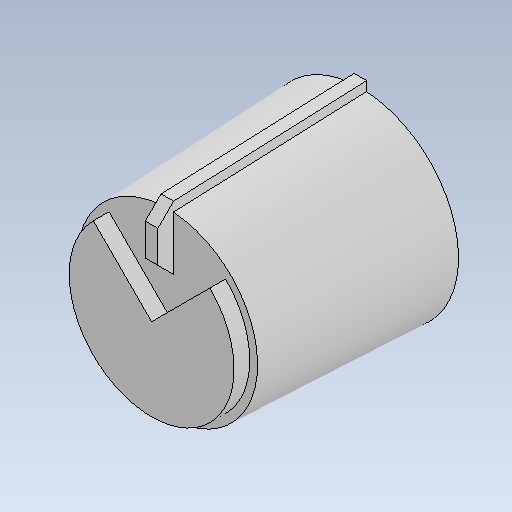
# Autodesk Inventor part: knob
Saved by Autodesk Inventor 2026.1 (Build 301233020, 233B)
## iProperties
Created: 2026-08-15
Part Number: knob
Material: 一般
Document SubType Name: Modeling
Designer: ug_nd
Density: 1 g/cm^3
Appearance: 既定
Author: ug_nd
Autodesk Inventor part; units mm, degrees
ref_plane "YZ Plane" through (0, 0, 0) normal (1, 0, 0) x (0, 1, 0)
ref_plane "XZ Plane" through (0, 0, 0) normal (0, 1, 0) x (-1, 0, 0)
ref_plane "XY Plane" through (0, 0, 0) normal (0, 0, 1) x (1, 0, 0)
sketch "スケッチ1" plane through (0, 0, 0) normal (1, 0, 0) x (0, 1, 0)
  line L0 (0, 0) -> (6.25, 0)
  line L1 (6.25, 0) -> (5.75, 12.3)
  line L2 (5.75, 12.3) -> (5.25, 12.3)
  line L3 (0, 13.3) -> (0, 0)
  line L4 (0, -2.66) -> (0, 15.96) construction
  line L5 (5.25, 12.3) -> (5.25, 13.3)
  line L6 (5.25, 13.3) -> (0, 13.3)
  dimension "d0" = 12.5
  dimension "d1" = 10.5
  dimension "d2" = 1
  dimension "d3" = 13.3
  dimension "d4" = 11.5
  constraints: 12 end point, 3 horizontal, 2 vertical, 2 other
  measures "d2" distance between parallel lines of L2 L6
  measures "d3" distance between parallel lines of L6 L0
revolve "回転1" add sketch "スケッチ1" angle 360 about axis through (0, 0, -10) along (0, 0, 1)
sketch "スケッチ2" plane through (0, 0, 13.3) normal (0, 0, 1) x (1, 0, 0)
  line L0 (0, -8.75) -> (0, 8.75) construction
  line L1 (0, 0) -> (3.7123, 3.7123)
  circle A0 centre (0, 0) radius 5.25 construction
  line L2 (0, 0) -> (-3.7123, 3.7123)
  arc A1 (3.7123, 3.7123) -> (-3.7123, 3.7123) centre (0, 0) ccw
  constraints: 4 end point, 2 point on circle, 1 centre point, 1 perpendicular, 1 symmetric about line, 3 other
extrude "押し出し1" cut sketch "スケッチ2" against normal up to surface (1 mm away)
sketch "スケッチ3" plane through (0, 0, 0) normal (1, 0, 0) x (0, 1, 0)
  line L0 (6.85, 0) -> (6.3093, 13.3)
  line L1 (6.3093, 13.3) -> (2.3093, 13.3)
  line L2 (6.25, 0) -> (-6.25, 0) construction
  line L3 (-6.25, 0) -> (-5.75, 12.3) construction
  line L4 (-5.75, 12.3) -> (-5.25, 12.3) construction
  line L5 (-5.25, 12.3) -> (-5.25, 13.3) construction
  line L6 (-5.25, 13.3) -> (0, 13.3) construction
  line L7 (0, 13.3) -> (0, 12.3) construction
  line L8 (0, 12.3) -> (5.75, 12.3) construction
  line L9 (5.75, 12.3) -> (6.25, 0) projected
  line L10 (6.85, 0) -> (6.25, 0)
  line L11 (2.3093, 13.3) -> (2.3093, 12.3)
  line L12 (5.75, 12.3) -> (2.3093, 12.3)
  line L13 (6.35, 12.3) -> (5.35, 13.3)
  line L14 (2.3093, 12.3) -> (3.3093, 13.3)
  point P0 (0, 0)
  dimension "d8" = 1
  dimension "d9" = 13.1
  dimension "d10" = 0.6
  dimension "d11" = 4
  dimension "d14" = 45
  constraints: 14 end point, 4 point on line, 2 horizontal, 2 perpendicular, 1 parallel, 1 vertical
  measures "d8" distance of L1.end L11.end
  measures "d9" distance of L2.end L0.start
  measures "d10" distance of L0.start L2.start
  measures "d11" distance of L0.end L1.end
  measures "d14" angle of L11 L14
extrude "押し出し2" add sketch "スケッチ3" along normal mid plane 0.8 contours L10 L9 L12 L14 L1 L13 L0
sketch "スケッチ4" plane through (0, 0, 0) normal (0, 0, 1) x (1, 0, 0)
  line L0 (1.5, 2.5981) -> (1.5, -2.5981)
  arc A0 (1.5, 2.5981) -> (1.5, -2.5981) centre (0, 0) ccw
  point P0 (-3, 0)
  dimension "d15" = 4.5
  dimension "d16" = 6
  constraints: 3 point on circle, 2 end point, 1 centre point, 1 coincident, 1 vertical
  measures "d15" distance from line of point (-3, 0) L0
  measures "d16" diameter of A0
extrude "押し出し3" cut sketch "スケッチ4" along normal blind 11
